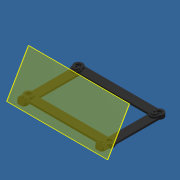
# Autodesk Inventor part: Moterboard_Mount
Saved by Autodesk Inventor 2014 SP2 (Build 180246200, 246)
## iProperties
Created: 2015-02-22
Part Number: Moterboard_Mount
Material: ABS-Kunststoff - Schwarz
Document SubType Name: Modeling
Designer: 4ndreas
Density: 1.06 g/cm^3
Appearance: Glatt - weiß(2)
Author: 4ndreas
Autodesk Inventor part; units mm, degrees
ref_plane "YZ Plane" through (0, 0, 0) normal (1, 0, 0) x (0, 1, 0)
ref_plane "XZ Plane" through (0, 0, 0) normal (0, 1, 0) x (-1, 0, 0)
ref_plane "XY Plane" through (0, 0, 0) normal (0, 0, 1) x (1, 0, 0)
sketch "Skizze1" plane through (0, 0, 0) normal (0, 0, 1) x (1, 0, 0)
  circle A0 centre (-65, -39.9989) radius 2 projected
  circle A1 centre (65, 40.0011) radius 2 projected
  circle A2 centre (65, -39.9989) radius 2 projected
  circle A3 centre (-65, 40.0011) radius 2 projected
  line L0 (-80, -49.9989) -> (-72, -49.9989) construction
  line L1 (-72, -49.9989) -> (-72, -60.3935) construction
  line L2 (-72, -60.3935) -> (72, -60.3935) construction
  line L3 (72, -60.3935) -> (72, -49.9989) construction
  line L4 (72, -49.9989) -> (80, -49.9989) construction
  line L5 (80, -49.9989) -> (80, 50.0011) construction
  line L6 (80, 50.0011) -> (72, 50.0011) construction
  line L7 (72, 50.0011) -> (72, 60.3935) construction
  line L8 (72, 60.3935) -> (-72, 60.3935) construction
  line L9 (-72, 60.3935) -> (-72, 50.0011) construction
  line L10 (-72, 50.0011) -> (-80, 50.0011) construction
  line L11 (-80, 50.0011) -> (-80, -49.9989) construction
  line L12 (65, -39.9989) -> (-65, -39.9989) construction
  line L13 (65, -32.9989) -> (-65, -32.9989)
  line L14 (-65, -46.9989) -> (65, -46.9989)
  arc A4 (65, -46.9989) -> (65, -32.9989) centre (65, -39.9989) ccw
  arc A5 (-65, -32.9989) -> (-65, -46.9989) centre (-65, -39.9989) ccw
  line L15 (65, 40.0011) -> (-65, 40.0011) construction
  line L16 (65, 47.0011) -> (-65, 47.0011)
  line L17 (-65, 33.0011) -> (65, 33.0011)
  arc A6 (65, 33.0011) -> (65, 47.0011) centre (65, 40.0011) ccw
  arc A7 (-65, 47.0011) -> (-65, 33.0011) centre (-65, 40.0011) ccw
  line L18 (-62.865, -50.7928) -> (62.865, -50.7928) construction
  line L19 (62.865, -50.7928) -> (62.865, 34.2972) construction
  line L20 (62.865, 34.2972) -> (-62.865, 34.2972) construction
  line L21 (-62.865, 34.2972) -> (-62.865, -50.7928) construction
  line L22 (0, -37.9989) -> (0, 40.0011) construction
  line L23 (-62.865, -50.7928) -> (-62.865, 40.0011) construction
  line L24 (-55.865, -50.7928) -> (-55.865, 40.0011)
  line L25 (-69.865, 40.0011) -> (-69.865, -50.7928)
  arc A8 (-69.865, -50.7928) -> (-55.865, -50.7928) centre (-62.865, -50.7928) ccw
  arc A9 (-55.865, 40.0011) -> (-69.865, 40.0011) centre (-62.865, 40.0011) ccw
  line L26 (62.865, -50.7928) -> (63, 40.0011) construction
  line L27 (69.865, -50.8032) -> (70, 39.9907)
  line L28 (56, 40.0115) -> (55.865, -50.7824)
  arc A10 (55.865, -50.7824) -> (69.865, -50.8032) centre (62.865, -50.7928) ccw
  arc A11 (70, 39.9907) -> (56, 40.0115) centre (63, 40.0011) ccw
  point P0 (0, 0)
  point P1 (0, -39.9989)
  point P2 (-62.865, -5.3958)
  point P3 (62.9325, -5.3958)
  dimension "d0" = 85.09
  dimension "d1" = 125.73
  constraints: 42 end point, 20 tangent, 16 point on circle, 8 centre point, 7 parallel, 4 midpoint, 3 perpendicular, 2 coincident, 2 point on line, 1 horizontal, 1 horizontal alignment, 2 other
  measures "d0" distance between parallel lines of L20 L18
  measures "d1" distance between parallel lines of L19 L21
extrude "Extrusion1" add sketch "Skizze1" along normal blind 3 contours A4 L27 L14 L28 L13 | L13 L28 L17 A6 L27 A4 | L28 L14 L24 L13 | A4 L27 | L24 L14 A5 L25 L13 | L13 A5 L25 A7 L17 L24 | L28 A11 L27 A6 L17 | L17 L24 A9 L16 A11 L28 | L14 A4 L27 A10 L28 | L27 A11 L16 A6 | L24 A8 L25 A5 L14 | L17 A7 L25 A9 L24 | L25 A5 | A7 L16 A9 L25
sketch "Skizze2" plane through (0, 0, 3) normal (0, 0, 1) x (1, 0, 0)
  arc A0 (-69.865, -50.7928) -> (-55.865, -50.7928) centre (-62.865, -50.7928) ccw projected
  arc A1 (55.865, -50.7824) -> (69.865, -50.8032) centre (62.865, -50.7928) ccw projected
  point P0 (0, 0)
  point P1 (62.865, 34.2972)
  point P2 (-62.865, 34.2972)
hole "Bohrung1" at (62.865, 34.2972, 3) at (-62.865, 34.2972, 3) at (-62.865, -50.7928, 3) at (62.865, -50.7928, 3) direction (0, 0, -1) diameter 3 end through all
sketch "Skizze3" plane through (0, 0, 3) normal (0, 0, 1) x (1, 0, 0)
  circle A0 centre (-62.865, -50.7928) radius 1.5 projected
  circle A1 centre (62.865, 34.2972) radius 1.5 projected
  circle A2 centre (-62.865, 34.2972) radius 1.5 projected
  circle A3 centre (62.865, -50.7928) radius 1.5 projected
  arc A4 (-69.865, -34.9658) -> (-69.865, -45.0319) centre (-65, -39.9989) ccw projected
  arc A5 (-69.865, -50.7928) -> (-55.865, -50.7928) centre (-62.865, -50.7928) ccw projected
  line L0 (-55.865, -46.9989) -> (55.8706, -46.9989) projected
  arc A6 (55.865, -50.7824) -> (69.865, -50.8032) centre (62.865, -50.7928) ccw projected
  arc A7 (69.8736, -45.0236) -> (69.8885, -34.9886) centre (65, -39.9989) ccw projected
  arc A8 (69.9927, 35.0947) -> (65, 47.0011) centre (65, 40.0011) ccw projected
  arc A9 (-65, 47.0011) -> (-69.865, 34.9681) centre (-65, 40.0011) ccw projected
  circle A10 centre (-65, 40.0011) radius 2 projected
  circle A11 centre (65, 40.0011) radius 2 projected
  circle A12 centre (-65, -39.9989) radius 2 projected
  circle A13 centre (65, -39.9989) radius 2 projected
  line L1 (-55.865, -32.9989) -> (-55.865, 33.0011) projected
  line L2 (-55.865, 33.0011) -> (55.9896, 33.0011) projected
  line L3 (55.9896, 33.0011) -> (55.8914, -32.9989) projected
  line L4 (-69.0415, -39.9989) -> (-67.0207, -36.4989)
  line L5 (-67.0207, -36.4989) -> (-62.9793, -36.4989)
  line L6 (-62.9793, -36.4989) -> (-60.9585, -39.9989)
  line L7 (-60.9585, -39.9989) -> (-62.9793, -43.4989)
  line L8 (-62.9793, -43.4989) -> (-67.0207, -43.4989)
  line L9 (-67.0207, -43.4989) -> (-69.0415, -39.9989)
  line L10 (-69.0415, 40.0011) -> (-67.0207, 43.5011)
  line L11 (-67.0207, 43.5011) -> (-62.9793, 43.5011)
  line L12 (-62.9793, 43.5011) -> (-60.9585, 40.0011)
  line L13 (-60.9585, 40.0011) -> (-62.9793, 36.5011)
  line L14 (-62.9793, 36.5011) -> (-67.0207, 36.5011)
  line L15 (-67.0207, 36.5011) -> (-69.0415, 40.0011)
  line L16 (69.0415, 40.0011) -> (67.0207, 36.5011)
  line L17 (67.0207, 36.5011) -> (62.9793, 36.5011)
  line L18 (62.9793, 36.5011) -> (60.9585, 40.0011)
  line L19 (60.9585, 40.0011) -> (62.9793, 43.5011)
  line L20 (62.9793, 43.5011) -> (67.0207, 43.5011)
  line L21 (67.0207, 43.5011) -> (69.0415, 40.0011)
  line L22 (69.0415, -39.9989) -> (67.0207, -43.4989)
  line L23 (67.0207, -43.4989) -> (62.9793, -43.4989)
  line L24 (62.9793, -43.4989) -> (60.9585, -39.9989)
  line L25 (60.9585, -39.9989) -> (62.9793, -36.4989)
  line L26 (62.9793, -36.4989) -> (67.0207, -36.4989)
  line L27 (67.0207, -36.4989) -> (69.0415, -39.9989)
  circle A14 centre (-65, -39.9989) radius 7
  circle A15 centre (65, -39.9989) radius 7
  arc A16 (-69.8355, 34.9397) -> (-58.0295, 39.3587) centre (-62.865, 34.2972) ccw
  arc A17 (-58.0295, 39.3587) -> (-69.8355, 34.9397) centre (-65, 40.0011) ccw
  arc A18 (69.7178, 34.8298) -> (58.0462, 39.1986) centre (65, 40.0011) ccw
  arc A19 (58.0462, 39.1986) -> (69.7178, 34.8298) centre (62.865, 34.2972) ccw
  circle A20 centre (-62.865, -50.7928) radius 7
  circle A21 centre (62.865, -50.7928) radius 7
  point P0 (0, 0)
  dimension "d11" = 7
  constraints: 48 end point, 12 coincident, 8 centre point, 8 point on circle, 4 concentric, 4 parallel, 4 tangent, 3 equal length, 52 other
  measures "d11" distance between parallel lines of L17 L20
sketch "Skizze4" plane through (0, 0, 3) normal (0, 0, 1) x (1, 0, 0)
  circle A0 centre (-62.865, -50.7928) radius 1.5 projected
  circle A1 centre (62.865, 34.2972) radius 1.5 projected
  circle A2 centre (-62.865, 34.2972) radius 1.5 projected
  circle A3 centre (62.865, -50.7928) radius 1.5 projected
  arc A4 (-69.865, -34.9658) -> (-69.865, -45.0319) centre (-65, -39.9989) ccw projected
  line L0 (-69.865, -45.0319) -> (-69.865, -50.7928) projected
  arc A5 (-69.865, -50.7928) -> (-55.865, -50.7928) centre (-62.865, -50.7928) ccw projected
  line L1 (-55.865, -50.7928) -> (-55.865, -46.9989) projected
  line L2 (-55.865, -46.9989) -> (55.8706, -46.9989) projected
  line L3 (55.8706, -46.9989) -> (55.865, -50.7824) projected
  arc A6 (55.865, -50.7824) -> (69.865, -50.8032) centre (62.865, -50.7928) ccw projected
  line L4 (69.865, -50.8032) -> (69.8736, -45.0236) projected
  arc A7 (69.8736, -45.0236) -> (69.8885, -34.9886) centre (65, -39.9989) ccw projected
  line L5 (69.8885, -34.9886) -> (69.9927, 35.0947) projected
  arc A8 (69.9927, 35.0947) -> (65, 47.0011) centre (65, 40.0011) ccw projected
  line L6 (65, 47.0011) -> (-65, 47.0011) projected
  arc A9 (-65, 47.0011) -> (-69.865, 34.9681) centre (-65, 40.0011) ccw projected
  line L7 (-69.865, 34.9681) -> (-69.865, -34.9658) projected
  circle A10 centre (-65, 40.0011) radius 2 projected
  circle A11 centre (65, 40.0011) radius 2 projected
  circle A12 centre (-65, -39.9989) radius 2 projected
  circle A13 centre (65, -39.9989) radius 2 projected
  line L8 (-55.865, -32.9989) -> (-55.865, 33.0011) projected
  line L9 (-55.865, 33.0011) -> (55.9896, 33.0011) projected
  line L10 (55.9896, 33.0011) -> (55.8914, -32.9989) projected
  line L11 (55.8914, -32.9989) -> (-55.865, -32.9989) projected
  point P0 (0, 0)
extrude "Extrusion2" add sketch "Skizze3" along normal blind 3 contours A14 A20 A4 | A20 A14 | A14 A20 A5 | A21 A15 A6 | A21 A15 | A15 A7 A21 | A18 A19 A8 | A17 A16 A9
sketch "Skizze5" plane through (0, 0, 6) normal (0, 0, 1) x (1, 0, 0)
  line L0 (67.0207, 36.5011) -> (62.9793, 36.5011) projected
  circle A0 centre (62.865, 34.2972) radius 1.5 projected
  arc A1 (58.0462, 39.1986) -> (69.7178, 34.8298) centre (62.865, 34.2972) ccw projected
  arc A2 (61.5434, 38.9881) -> (67.2117, 36.5011) centre (62.865, 34.2972) ccw
  line L1 (-67.0207, 43.5011) -> (-62.9793, 43.5011) projected
  line L2 (-62.9793, 43.5011) -> (-60.9585, 40.0011) projected
  line L3 (-60.9585, 40.0011) -> (-62.9793, 36.5011) projected
  line L4 (-62.9793, 36.5011) -> (-67.0207, 36.5011) projected
  line L5 (-67.0207, 36.5011) -> (-69.0415, 40.0011) projected
  line L6 (-69.0415, 40.0011) -> (-67.0207, 43.5011) projected
  circle A3 centre (-62.865, 34.2972) radius 1.5 projected
  arc A4 (-69.8355, 34.9397) -> (-58.0295, 39.3587) centre (-62.865, 34.2972) ccw projected
  arc A5 (-58.0295, 39.3587) -> (-69.8355, 34.9397) centre (-65, 40.0011) ccw projected
  circle A6 centre (62.865, -50.7928) radius 1.5 projected
  line L7 (67.0207, -43.4989) -> (62.9793, -43.4989) projected
  line L8 (62.9793, -43.4989) -> (60.9585, -39.9989) projected
  line L9 (60.9585, -39.9989) -> (62.9793, -36.4989) projected
  line L10 (62.9793, -36.4989) -> (67.0207, -36.4989) projected
  line L11 (67.0207, -36.4989) -> (69.0415, -39.9989) projected
  line L12 (69.0415, -39.9989) -> (67.0207, -43.4989) projected
  arc A7 (68.1784, -46.2357) -> (59.6866, -44.556) centre (65, -39.9989) ccw projected
  arc A8 (59.6866, -44.556) -> (68.1784, -46.2357) centre (62.865, -50.7928) ccw projected
  circle A9 centre (-62.865, -50.7928) radius 1.5 projected
  line L13 (-67.0207, -36.4989) -> (-62.9793, -36.4989) projected
  line L14 (-62.9793, -36.4989) -> (-60.9585, -39.9989) projected
  line L15 (-60.9585, -39.9989) -> (-62.9793, -43.4989) projected
  line L16 (-62.9793, -43.4989) -> (-67.0207, -43.4989) projected
  line L17 (-67.0207, -43.4989) -> (-69.0415, -39.9989) projected
  line L18 (-69.0415, -39.9989) -> (-67.0207, -36.4989) projected
  arc A10 (-59.6866, -44.556) -> (-68.1784, -46.2357) centre (-65, -39.9989) ccw projected
  arc A11 (-68.1784, -46.2357) -> (-59.6866, -44.556) centre (-62.865, -50.7928) ccw projected
  circle A12 centre (62.865, -50.7928) radius 5
  circle A13 centre (-62.865, -50.7928) radius 5
  arc A14 (-67.3531, 36.5011) -> (-61.4782, 39.101) centre (-62.865, 34.2972) ccw
  line L19 (-62.9793, 36.5011) -> (-67.0207, 36.5011) projected
  line L20 (-62.9793, 36.5011) -> (-67.3531, 36.5011)
  line L21 (-61.4782, 39.101) -> (-62.9793, 36.5011)
  line L22 (61.5434, 38.9881) -> (62.9793, 36.5011)
  line L23 (62.9793, 36.5011) -> (67.2117, 36.5011)
  point P0 (0, 0)
  dimension "d14" = 2
  dimension "d15" = 2
  dimension "d16" = 2
  constraints: 8 end point, 5 point on circle, 4 centre point, 4 coincident, 3 point on line, 2 collinear, 2 parallel, 1 equal radius
  measures "d14" radial gap between concentric circles of A2 A1
  measures "d15" radial gap between concentric circles of A14 A4
  measures "d16" radial gap between concentric circles of A13 A11
extrude "Extrusion3" add sketch "Skizze5" along normal blind 2 contours L23 A2 L22 L0 | L4 L3 A14 L20 | A12 | A13
sketch "Skizze6" plane through (69.9927, 35.0947, 3) normal (0.9999989, -0.0014869, 0) x (0, 0, -1)
  line L0 (3, 0) -> (0, 0) projected
  line L1 (0, -70.0834) -> (0, 0) projected
  line L2 (0, -70.0834) -> (3, -70.0834) projected
  line L3 (3, -70.0834) -> (3, 0) projected
  line L4 (-8.8106, -86.2661) -> (3, -93.085)
  line L5 (3, -86.0746) -> (3, -93.085) projected
  point P0 (3, -35.1988)
  point P1 (3, -86.0954)
  dimension "d22" = 60
  constraints: 2 end point
  measures "d22" angle of L4 L3
ref_plane "Arbeitsebene1" through (69.8644, -51.1713, 11.8106) normal (-0.0012877, -0.8660244, 0.5) x (-0.0007434, -0.4999994, -0.8660254)
ref_plane "Arbeitsebene2" through (69.8657, -50.3052, 11.3106) normal (-0.0012877, -0.8660244, 0.5) x (-0.0007434, -0.4999994, -0.8660254)
split "Trennen2" plane through (69.8657, -50.3052, 11.3106) removes the side toward (-0.0012877, -0.8660244, 0.5)
